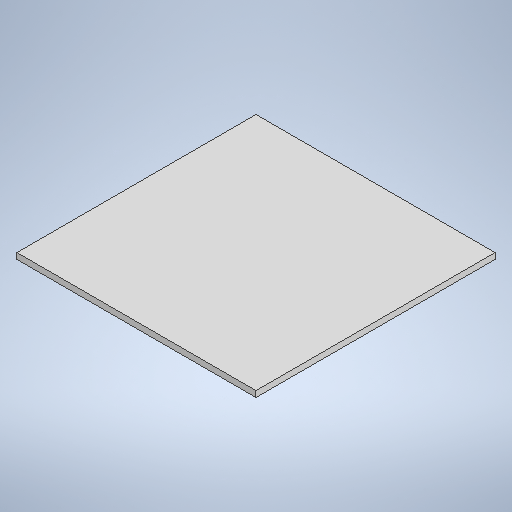
# Autodesk Inventor part: Acrylic top
Saved by Autodesk Inventor 2025.2 (Build 292293000, 293)
## iProperties
Created: 2025-03-13
Part Number: Acrylic top
Material: Generic
Document SubType Name: Modeling
Designer: CZ
Density: 1 g/cm^3
Appearance: Default
Author: CZ
Autodesk Inventor part; units mm, degrees
ref_plane "YZ Plane" through (0, 0, 0) normal (1, 0, 0) x (0, 1, 0)
ref_plane "XZ Plane" through (0, 0, 0) normal (0, 1, 0) x (-1, 0, 0)
ref_plane "XY Plane" through (0, 0, 0) normal (0, 0, 1) x (1, 0, 0)
sketch "Sketch1" plane through (0, 0, 0) normal (0, 1, 0) x (-1, 0, 0)
  line L0 (80, 80) -> (-80, 80)
  line L1 (-80, 80) -> (-80, -80)
  line L2 (-80, -80) -> (80, -80)
  line L3 (80, -80) -> (80, 80)
  point P0 (0, 0)
  point P1 (0, -80)
  dimension "d0" = 160
  dimension "d1" = 80
  dimension "d2" = 160
  dimension "d3" = 80
  constraints: 8 end point, 2 parallel, 1 horizontal, 1 midpoint, 1 perpendicular
  measures "d0" distance from line of point (0, -80) L0
  measures "d1" distance from line of point (0, 0) L2
  measures "d2" distance between parallel lines of L1 L3
  measures "d3" distance from line of point (0, 0) L3
extrude "Extrusion1" add sketch "Sketch1" along normal blind 4
body "Solid1"
